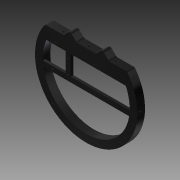
# Autodesk Inventor part: Middle Plate
Saved by Autodesk Inventor 2015 (Build 190159000, 159)
## iProperties
Created: 2016-02-10
Part Number: Middle Plate
Material: ABS Plastic
Document SubType Name: Modeling
Designer: James
Density: 1.06 g/cm^3
Appearance: Smooth - White
Author: James
Autodesk Inventor part; units mm, degrees
ref_plane "YZ Plane" through (0, 0, 0) normal (1, 0, 0) x (0, 1, 0)
ref_plane "XZ Plane" through (0, 0, 0) normal (0, 1, 0) x (-1, 0, 0)
ref_plane "XY Plane" through (0, 0, 0) normal (0, 0, 1) x (1, 0, 0)
sketch "Sketch1" plane through (0, 0, 0) normal (0, 1, 0) x (-1, 0, 0)
  line L0 (0, 45) -> (69.282, 45)
  line L1 (0, 45) -> (-69.282, 45)
  arc A0 (-73.6122, 42.5) -> (73.6122, 42.5) centre (0, 0) ccw
  arc A1 (-81.5365, 57.8947) -> (81.5365, 57.8947) centre (0, 0) ccw
  arc A2 (73.6122, 42.5) -> (69.282, 45) centre (69.282, 40) ccw
  arc A3 (-69.282, 45) -> (-73.6122, 42.5) centre (-69.282, 40) ccw
  arc A4 (-77.4597, 60) -> (-81.5365, 57.8947) centre (-77.4597, 55) ccw
  arc A5 (81.5365, 57.8947) -> (77.4597, 60) centre (77.4597, 55) ccw
  line L2 (0, 0) -> (-65.4074, -65.4074) construction
  line L3 (0, 0) -> (65.4074, -65.4074) construction
  circle A6 centre (-65.4074, -65.4074) radius 1.6
  circle A7 centre (65.4074, -65.4074) radius 1.6
  circle A8 centre (-31.5451, 65.2705) radius 1.6
  circle A9 centre (31.5451, 65.2705) radius 1.6
  line L4 (-31.5451, 65.2705) -> (-24.0451, 65.2705) construction
  line L5 (-28.0096, 69.235) -> (-20.2391, 61.4645)
  line L6 (-35.0806, 69.235) -> (-42.8511, 61.4645)
  line L7 (35.0806, 69.235) -> (42.8511, 61.4645)
  line L8 (28.0096, 69.235) -> (20.2391, 61.4645)
  line L9 (46.3867, 60) -> (77.4597, 60)
  line L10 (16.7035, 60) -> (-16.7035, 60)
  line L11 (-46.3867, 60) -> (-77.4597, 60)
  arc A10 (-46.3867, 60) -> (-42.8511, 61.4645) centre (-46.3867, 65) ccw
  arc A11 (-28.0096, 69.235) -> (-35.0806, 69.235) centre (-31.5451, 65.6994) ccw
  arc A12 (-20.2391, 61.4645) -> (-16.7035, 60) centre (-16.7035, 65) ccw
  arc A13 (16.7035, 60) -> (20.2391, 61.4645) centre (16.7035, 65) ccw
  arc A14 (35.0806, 69.235) -> (28.0096, 69.235) centre (31.5451, 65.6994) ccw
  arc A15 (42.8511, 61.4645) -> (46.3867, 60) centre (46.3867, 65) ccw
  point P0 (80, 60)
  point P1 (-80, 60)
  point P2 (72.111, 45)
  point P3 (-72.111, 45)
  point P4 (-31.5451, 72.7705)
  point P5 (31.5451, 72.7705)
  dimension "d23" = 5
  dimension "d24" = 5
  dimension "d28" = 3.2
  dimension "d29" = 3.2
  dimension "d34" = 3.2
  dimension "d35" = 7.5
  dimension "d37" = 7.5
  dimension "d38" = 5
  constraints: 28 point on circle, 24 end point, 18 tangent, 16 centre point, 7 equal radius, 7 point on line, 5 coincident, 2 collinear, 2 horizontal, 2 perpendicular
  measures "d23" radius of A2
  measures "d24" radius of A3
  measures "d28" diameter of A6
  measures "d29" diameter of A7
  measures "d34" diameter of A8
  measures "d35" distance of L4.start point (-31.545, 72.77)
  measures "d37" distance of A9.centre point (31.545, 72.77)
  measures "d38" radius of A10
extrude "Extrusion1" add sketch "Sketch1" along normal blind 15
sketch "Sketch3" plane through (0, 15, 0) normal (0, 1, 0) x (1, 0, 0)
  arc A0 (-73.6122, -42.5) -> (-69.282, -45) centre (-69.282, -40) ccw projected
  arc A1 (73.6122, -42.5) -> (-73.6122, -42.5) centre (0, 0) ccw projected
  arc A2 (69.282, -45) -> (73.6122, -42.5) centre (69.282, -40) ccw projected
  line L0 (69.282, -45) -> (-69.282, -45) projected
  circle A3 centre (-31.5451, -65.2705) radius 1.6 projected
  circle A4 centre (31.5451, -65.2705) radius 1.6 projected
  circle A5 centre (-65.4074, 65.4074) radius 1.6 projected
  circle A6 centre (65.4074, 65.4074) radius 1.6 projected
  arc A7 (77.4597, -60) -> (81.5365, -57.8947) centre (77.4597, -55) ccw projected
  arc A8 (81.5365, -57.8947) -> (-81.5365, -57.8947) centre (0, 0) ccw projected
  arc A9 (-81.5365, -57.8947) -> (-77.4597, -60) centre (-77.4597, -55) ccw projected
  line L1 (-77.4597, -60) -> (-46.3867, -60) projected
  arc A10 (-42.8511, -61.4645) -> (-46.3867, -60) centre (-46.3867, -65) ccw projected
  line L2 (-42.8511, -61.4645) -> (-35.0806, -69.235) projected
  arc A11 (-35.0806, -69.235) -> (-28.0096, -69.235) centre (-31.5451, -65.6994) ccw projected
  line L3 (-28.0096, -69.235) -> (-20.2391, -61.4645) projected
  arc A12 (-16.7035, -60) -> (-20.2391, -61.4645) centre (-16.7035, -65) ccw projected
  line L4 (-16.7035, -60) -> (16.7035, -60) projected
  arc A13 (20.2391, -61.4645) -> (16.7035, -60) centre (16.7035, -65) ccw projected
  line L5 (20.2391, -61.4645) -> (28.0096, -69.235) projected
  arc A14 (28.0096, -69.235) -> (35.0806, -69.235) centre (31.5451, -65.6994) ccw projected
  line L6 (35.0806, -69.235) -> (42.8511, -61.4645) projected
  arc A15 (46.3867, -60) -> (42.8511, -61.4645) centre (46.3867, -65) ccw projected
  line L7 (46.3867, -60) -> (77.4597, -60) projected
  line L8 (-16.7035, -60) -> (16.7035, -60) projected
  line L9 (69.282, -45) -> (-69.282, -45) projected
  line L10 (-5.2, -55) -> (-5.2, -50.6)
  line L11 (-5.2, -50.6) -> (5.2, -50.6)
  line L12 (5.2, -50.6) -> (5.2, -55)
  arc A16 (-2.5852, -55) -> (0.0053, -56.8093) centre (-0.0011, -54.0593) ccw
  arc A17 (0.0053, -56.8093) -> (2.583, -55) centre (-0.0011, -54.0593) ccw
  line L13 (5.2, -55) -> (2.583, -55)
  line L14 (-5.2, -55) -> (-2.5852, -55)
  line L15 (42.9967, -58.2699) -> (40.7967, -54.4594)
  line L16 (40.7967, -54.4594) -> (49.8033, -49.2594)
  line L17 (49.8033, -49.2594) -> (52.0033, -53.0699)
  arc A18 (45.2611, -56.9625) -> (48.4093, -57.2341) centre (47.0287, -54.8557) ccw
  arc A19 (48.4093, -57.2341) -> (49.7369, -54.3784) centre (47.0287, -54.8557) ccw
  line L18 (52.0033, -53.0699) -> (49.7369, -54.3784)
  line L19 (42.9967, -58.2699) -> (45.2611, -56.9625)
  line L20 (79.6724, -52.0033) -> (75.8619, -49.8033)
  line L21 (75.8619, -49.8033) -> (81.0619, -40.7967)
  line L22 (81.0619, -40.7967) -> (84.8724, -42.9967)
  arc A20 (80.9798, -49.7389) -> (83.842, -48.4) centre (81.4572, -47.0306) ccw
  arc A21 (83.842, -48.4) -> (83.5639, -45.2631) centre (81.4572, -47.0306) ccw
  line L23 (84.8724, -42.9967) -> (83.5639, -45.2631)
  line L24 (79.6724, -52.0033) -> (80.9798, -49.7389)
  line L25 (95, -5.2) -> (90.6, -5.2)
  line L26 (90.6, -5.2) -> (90.6, 5.2)
  line L27 (90.6, 5.2) -> (95, 5.2)
  arc A22 (95, -2.5852) -> (96.8093, 0.0053) centre (94.0593, -0.0011) ccw
  arc A23 (96.8093, 0.0053) -> (95, 2.583) centre (94.0593, -0.0011) ccw
  line L28 (95, 5.2) -> (95, 2.583)
  line L29 (95, -5.2) -> (95, -2.5852)
  line L30 (84.8724, 42.9967) -> (81.0619, 40.7967)
  line L31 (81.0619, 40.7967) -> (75.8619, 49.8033)
  line L32 (75.8619, 49.8033) -> (79.6724, 52.0033)
  arc A24 (83.565, 45.2611) -> (83.8366, 48.4093) centre (81.4583, 47.0287) ccw
  arc A25 (83.8366, 48.4093) -> (80.9809, 49.7369) centre (81.4583, 47.0287) ccw
  line L33 (79.6724, 52.0033) -> (80.9809, 49.7369)
  line L34 (84.8724, 42.9967) -> (83.565, 45.2611)
  line L35 (52.0033, 79.6724) -> (49.8033, 75.8619)
  line L36 (49.8033, 75.8619) -> (40.7967, 81.0619)
  line L37 (40.7967, 81.0619) -> (42.9967, 84.8724)
  arc A26 (49.7389, 80.9798) -> (48.4, 83.842) centre (47.0306, 81.4572) ccw
  arc A27 (48.4, 83.842) -> (45.2631, 83.5639) centre (47.0306, 81.4572) ccw
  line L38 (42.9967, 84.8724) -> (45.2631, 83.5639)
  line L39 (52.0033, 79.6724) -> (49.7389, 80.9798)
  line L40 (5.2, 95) -> (5.2, 90.6)
  line L41 (5.2, 90.6) -> (-5.2, 90.6)
  line L42 (-5.2, 90.6) -> (-5.2, 95)
  arc A28 (2.5852, 95) -> (-0.0053, 96.8093) centre (0.0011, 94.0593) ccw
  arc A29 (-0.0053, 96.8093) -> (-2.583, 95) centre (0.0011, 94.0593) ccw
  line L43 (-5.2, 95) -> (-2.583, 95)
  line L44 (5.2, 95) -> (2.5852, 95)
  line L45 (-42.9967, 84.8724) -> (-40.7967, 81.0619)
  line L46 (-40.7967, 81.0619) -> (-49.8033, 75.8619)
  line L47 (-49.8033, 75.8619) -> (-52.0033, 79.6724)
  arc A30 (-45.2611, 83.565) -> (-48.4093, 83.8366) centre (-47.0287, 81.4583) ccw
  arc A31 (-48.4093, 83.8366) -> (-49.7369, 80.9809) centre (-47.0287, 81.4583) ccw
  line L48 (-52.0033, 79.6724) -> (-49.7369, 80.9809)
  line L49 (-42.9967, 84.8724) -> (-45.2611, 83.565)
  line L50 (-79.6724, 52.0033) -> (-75.8619, 49.8033)
  line L51 (-75.8619, 49.8033) -> (-81.0619, 40.7967)
  line L52 (-81.0619, 40.7967) -> (-84.8724, 42.9967)
  arc A32 (-80.9798, 49.7389) -> (-83.842, 48.4) centre (-81.4572, 47.0306) ccw
  arc A33 (-83.842, 48.4) -> (-83.5639, 45.2631) centre (-81.4572, 47.0306) ccw
  line L53 (-84.8724, 42.9967) -> (-83.5639, 45.2631)
  line L54 (-79.6724, 52.0033) -> (-80.9798, 49.7389)
  line L55 (-95, 5.2) -> (-90.6, 5.2)
  line L56 (-90.6, 5.2) -> (-90.6, -5.2)
  line L57 (-90.6, -5.2) -> (-95, -5.2)
  arc A34 (-95, 2.5852) -> (-96.8093, -0.0053) centre (-94.0593, 0.0011) ccw
  arc A35 (-96.8093, -0.0053) -> (-95, -2.583) centre (-94.0593, 0.0011) ccw
  line L58 (-95, -5.2) -> (-95, -2.583)
  line L59 (-95, 5.2) -> (-95, 2.5852)
  line L60 (-84.8724, -42.9967) -> (-81.0619, -40.7967)
  line L61 (-81.0619, -40.7967) -> (-75.8619, -49.8033)
  line L62 (-75.8619, -49.8033) -> (-79.6724, -52.0033)
  arc A36 (-83.565, -45.2611) -> (-83.8366, -48.4093) centre (-81.4583, -47.0287) ccw
  arc A37 (-83.8366, -48.4093) -> (-80.9809, -49.7369) centre (-81.4583, -47.0287) ccw
  line L63 (-79.6724, -52.0033) -> (-80.9809, -49.7369)
  line L64 (-84.8724, -42.9967) -> (-83.565, -45.2611)
  line L65 (-52.0033, -53.0699) -> (-49.8033, -49.2594)
  line L66 (-49.8033, -49.2594) -> (-40.7967, -54.4594)
  line L67 (-40.7967, -54.4594) -> (-42.9967, -58.2699)
  arc A38 (-49.7389, -54.3773) -> (-48.4, -57.2394) centre (-47.0306, -54.8546) ccw
  arc A39 (-48.4, -57.2394) -> (-45.2631, -56.9614) centre (-47.0306, -54.8546) ccw
  line L68 (-42.9967, -58.2699) -> (-45.2631, -56.9614)
  line L69 (-52.0033, -53.0699) -> (-49.7389, -54.3773)
  line L70 (46.3867, -60) -> (77.4597, -60) projected
  line L71 (-77.4597, -60) -> (-46.3867, -60) projected
  line L72 (0.0053, -56.8093) -> (0, -60)
  point P0 (86.6025, -50)
  point P1 (100, 0)
  point P2 (86.6025, 50)
  point P3 (50, 86.6025)
  point P4 (0, 100)
  point P5 (-50, 86.6025)
  point P6 (-86.6025, 50)
  point P7 (-100, 0)
  point P8 (-86.6025, -50)
  dimension "d48" = 360
  constraints: 122 end point, 48 point on circle, 24 centre point, 12 coincident, 1 midpoint, 135 other
extrude "Extrusion3" cut sketch "Sketch3" against normal blind 13 contours L10 L11 L12 L13 A17 A16 L14 | L15 L16 L17 L18 A19 A18 L19 | L20 L21 L22 L23 A21 A20 L24 | L25 L26 L27 L28 A23 A22 L29 | L30 L31 L32 L33 A25 A24 L34 | L35 L36 L37 L38 A27 A26 L39 | L40 L41 L42 L43 A29 A28 L44 | L45 L46 L47 L48 A31 A30 L49 | L50 L51 L52 L53 A33 A32 L54 | L55 L56 L57 L58 A35 A34 L59 | L60 L61 L62 L63 A37 A36 L64 | L65 L66 L67 L68 A39 A38 L69
sketch "Sketch4" plane through (-5.2, 15, 50.6) normal (0, 0, 1) x (1, 0, 0)
  line L0 (0, 0) -> (10.4, 0) projected
  line L1 (5.2, 0) -> (5.2, -9.5)
  circle A0 centre (5.2, -9.5) radius 1.5
  point P0 (5.2, -15)
  dimension "d52" = 9.5
  dimension "d53" = 3
  constraints: 2 end point, 1 centre point, 1 coincident, 1 midpoint, 1 vertical
  measures "d52" distance of L1.start L1.end
  measures "d53" diameter of A0
extrude "Extrusion4" cut sketch "Sketch4" along normal through all
sketch "Sketch5" plane through (40.7967, 2, 54.4594) normal (0.5, 0, 0.8660254) x (0.8660254, 0, -0.5)
  line L0 (0, 13) -> (10.4, 13) projected
  line L1 (5.2, 13) -> (5.2, 3.5)
  circle A0 centre (5.2, 3.5) radius 1.5
  point P0 (-8.1013, -2)
  dimension "d56" = 9.5
  dimension "d57" = 3
  constraints: 2 end point, 1 centre point, 1 coincident, 1 midpoint, 1 vertical
  measures "d56" distance of L1.start L1.end
  measures "d57" diameter of A0
extrude "Extrusion5" cut sketch "Sketch5" along normal through all
sketch "Sketch6" plane through (75.8619, 2, 49.8033) normal (0.8660254, 0, 0.5) x (0.5, 0, -0.8660254)
  line L0 (0, 13) -> (10.4, 13) projected
  line L1 (5.2, 13) -> (5.2, 3.5)
  line L2 (5.2, 13) -> (14.7, 13) construction
  circle A0 centre (5.2, 3.5) radius 1.5
  point P0 (5.2, -2)
  dimension "d60" = 9.5
  dimension "d61" = 90
  dimension "d62" = 3
  constraints: 4 end point, 1 centre point, 1 coincident, 1 horizontal, 1 midpoint, 1 perpendicular, 1 vertical
  measures "d60" distance of L1.start L1.end
  measures "d61" angle of L1 L2
  measures "d62" diameter of A0
extrude "Extrusion6" cut sketch "Sketch6" along normal through all
pattern_circular "Circular Pattern1" count 9 over 240 about axis through (0, -10, 0) along (0, 1, 0) of "Extrusion6"
sketch "Sketch7" plane through (-49.8033, 2, 49.2594) normal (-0.5, 0, 0.8660254) x (0.8660254, 0, 0.5)
  line L0 (0, 13) -> (10.4, 13) projected
  line L1 (5.2, 13) -> (5.2, 3.5)
  circle A0 centre (5.2, 3.5358) radius 1.5
  point P0 (18.5013, -2)
  dimension "d68" = 9.5
  dimension "d69" = 3
  constraints: 2 end point, 1 centre point, 1 midpoint, 1 point on line, 1 vertical
  measures "d68" distance of L1.start L1.end
  measures "d69" diameter of A0
extrude "Extrusion7" cut sketch "Sketch7" along normal through all
sketch "Sketch8" plane through (0, 0, 0) normal (0, -1, 0) x (1, 0, 0)
  line L0 (69.282, 45) -> (-69.282, 45)
  line L1 (0, 35) -> (77.4597, 35)
  line L2 (-83.565, 45.2611) -> (-84.8724, 42.9967)
  line L3 (-84.8724, 42.9967) -> (-81.0619, 40.7967) projected
  line L4 (-81.0619, 40.7967) -> (-75.8619, 49.8033)
  line L5 (-75.8619, 49.8033) -> (-79.6724, 52.0033)
  line L6 (-79.6724, 52.0033) -> (-80.9809, 49.7369)
  arc A0 (-80.9809, 49.7369) -> (-83.565, 45.2611) centre (-81.4583, 47.0287) ccw
  line L7 (80.9798, 49.7389) -> (79.6724, 52.0033)
  line L8 (79.6724, 52.0033) -> (75.8619, 49.8033)
  line L9 (75.8619, 49.8033) -> (81.0619, 40.7967)
  line L10 (81.0619, 40.7967) -> (84.8724, 42.9967) projected
  line L11 (84.8724, 42.9967) -> (83.5639, 45.2631)
  arc A1 (83.5639, 45.2631) -> (80.9798, 49.7389) centre (81.4572, 47.0306) ccw
  line L12 (-5.2, 50.6) -> (5.2, 50.6)
  line L13 (95, 2.5852) -> (95, 5.2) projected
  line L14 (95, 5.2) -> (90.6, 5.2) projected
  line L15 (90.6, 5.2) -> (90.6, -5.2) projected
  line L16 (90.6, -5.2) -> (95, -5.2) projected
  line L17 (95, -5.2) -> (95, -2.583) projected
  arc A2 (95, -2.583) -> (95, 2.5852) centre (94.0593, 0.0011) ccw projected
  line L18 (-95, -2.5852) -> (-95, -5.2) projected
  line L19 (-95, -5.2) -> (-90.6, -5.2) projected
  line L20 (-90.6, -5.2) -> (-90.6, 5.2) projected
  line L21 (-90.6, 5.2) -> (-95, 5.2) projected
  line L22 (-95, 5.2) -> (-95, 2.583) projected
  arc A3 (-95, 2.583) -> (-95, -2.5852) centre (-94.0593, -0.0011) ccw projected
  arc A4 (-69.282, 45) -> (-73.6122, 42.5) centre (-69.282, 40) ccw
  arc A5 (73.6122, 42.5) -> (69.282, 45) centre (69.282, 40) ccw
  line L23 (69.282, 45) -> (-69.282, 45)
  circle A6 centre (-35.1606, -3.1436) radius 1.6079
  circle A7 centre (16.8699, -8.2218) radius 1.6079
  circle A8 centre (15.6003, 40) radius 1.6079
  circle A9 centre (-35.1606, 24.7654) radius 1.6079
  circle A10 centre (-59.282, 40) radius 1.6079
  circle A11 centre (-65.6086, -8.2218) radius 1.6079
  line L24 (-65.6086, -3.2218) -> (-84.9389, -3.2218)
  line L25 (-65.6086, -13.2218) -> (-83.9654, -13.2218)
  line L26 (-83.9654, -13.2218) -> (83.9654, -13.2218)
  line L27 (-65.6086, -3.2218) -> (-40.1606, -3.2218)
  line L28 (-40.1606, -3.2218) -> (-40.1606, 35)
  line L29 (0, 35) -> (-30.1606, 35)
  line L30 (-40.1606, 35) -> (-77.4597, 35)
  line L31 (16.8699, -3.2218) -> (84.9389, -3.2218)
  line L32 (84.9389, -3.2218) -> (-30.1606, -3.2218)
  line L33 (-30.1606, 35) -> (-30.1606, -3.2218)
  arc A12 (83.9654, -13.2218) -> (84.9389, -3.2218) centre (0, 0) ccw
  arc A13 (77.4597, 35) -> (73.6122, 42.5) centre (0, 0) ccw
  arc A14 (-84.9389, -3.2218) -> (-83.9654, -13.2218) centre (0, 0) ccw
  arc A15 (-73.6122, 42.5) -> (-77.4597, 35) centre (0, 0) ccw
  arc A16 (-73.6122, 42.5) -> (73.6122, 42.5) centre (0, 0) ccw projected
  constraints: 44 end point, 20 centre point, 20 point on circle, 4 coincident, 2 vertical, 1 horizontal, 1 point on line
extrude "Extrusion9" add sketch "Sketch8" against normal blind 5 contours A5 A13 L1 L29 L33 L32 L31 A12 L26 L25 A14 L24 L27 L28 L30 A15 A4 L0
body "Solid1"
